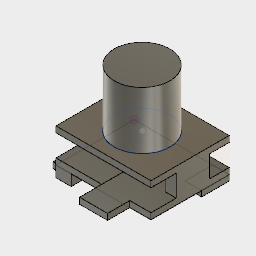
fx805 (Autodesk Fusion 360 design; units mm, degrees)
Autodesk Fusion 360 part; units mm, degrees
sketch "body2" plane through (0, 0, 0) normal (0, 0, 1) x (1, 0, 0)
  line L0 (0, 0) -> (17.1, 0)
  line L1 (17.1, 0) -> (17.1, -14.1)
  line L2 (17.1, -14.1) -> (0, -14.1)
  line L3 (0, -14.1) -> (0, 0)
  line L4 (17.1, 0) -> (14.1, 0)
  line L5 (14.1, 0) -> (14.1, -5)
  line L6 (14.1, -5) -> (17.1, -5)
  line L7 (17.1, -5) -> (17.1, 0)
  dimension "d1" = 17.1
  dimension "d2" = 14.1
  dimension "d19" = 5
  dimension "d20" = 3
  measures "d1" distance of L0.start L0.end
  measures "d2" distance of L0.start L2.end
  measures "d19" distance of L0.end L6.end
  measures "d20" distance of L0.end L4.end
extrude "Extrude1" add sketch "body2" along normal blind 6.1 makes body 1
sketch "body with camera" plane through (0, 0, 6.1) normal (0, 0, 1) x (-1, 0, 0)
  line L0 (0, 14.1) -> (-17.1, 14.1)
  line L1 (-17.1, 14.1) -> (-17.1, 0)
  line L2 (-17.1, 0) -> (0, 0)
  line L3 (0, 0) -> (0, 14.1)
  circle A0 centre (-8.55, 7.1407) radius 5
  dimension "d5" = 10
  measures "d5" diameter of A0
extrude "Extrude2" add sketch "body with camera" along normal blind 10.3 contours A0 bodies 1
sketch "body" plane through (0, 0, 0) normal (0, 0, -1) x (1, 0, 0)
  line L0 (17.1, 14.1) -> (0, 14.1)
  line L1 (0, 14.1) -> (0, 0)
  line L2 (0, 0) -> (17.1, 0)
  line L3 (17.1, 0) -> (17.1, 14.1)
  line L4 (0, 14.1) -> (2.75, 14.1)
  line L5 (2.75, 14.1) -> (2.75, 9.1)
  line L6 (2.75, 9.1) -> (0, 9.1)
  line L7 (0, 9.1) -> (0, 14.1)
  dimension "d8" = 5
  dimension "d9" = 2.75
  measures "d8" distance of L0.end L6.end
  measures "d9" distance of L0.end L4.end
extrude "Extrude3" add sketch "body" along normal blind 2 contours L0 L1 L4 L5 L6 L7 bodies 1
sketch "Sketch6" plane through (0, 0, 0) normal (0, 1, 0) x (-1, 0, 0)
  line L0 (-17.1, 0) -> (0, 0)
  line L1 (0, 0) -> (0, 6.1)
  line L2 (0, 6.1) -> (-17.1, 6.1)
  line L3 (-17.1, 6.1) -> (-17.1, 0)
sketch "Sketch7" plane through (0, 0, 0) normal (-1, 0, 0) x (0, -1, 0)
  line L0 (14.1, -2) -> (14.1, 6.1)
  line L1 (14.1, 6.1) -> (0, 6.1)
  line L2 (0, 6.1) -> (0, 0)
  line L3 (0, 0) -> (9.1, 0)
  line L4 (9.1, 0) -> (9.1, -2)
  line L5 (9.1, -2) -> (14.1, -2)
  line L6 (9.7769, -1.5456) -> (13.3769, -1.5456)
  line L7 (13.3769, -1.5456) -> (13.3769, -0.4527)
  line L8 (13.3769, -0.4527) -> (9.7769, -0.4527)
  line L9 (9.7769, -0.4527) -> (9.7769, -1.5456)
  line L10 (9.7769, -1.5456) -> (13.3769, -0.4527) construction
  line L11 (13.3769, -1.5456) -> (9.7769, -0.4527) construction
  point P0 (11.5769, -0.9991)
extrude "Extrude4" add sketch "Sketch7" along normal blind 1.25 contours L6 L7 L8 L9 bodies 1
sketch "Sketch8" plane through (0, -14.1, 0) normal (0, -1, 0) x (1, 0, 0)
  line L0 (2.75, 0) -> (17.1, 0)
  line L1 (17.1, 0) -> (17.1, 6.1)
  line L2 (17.1, 6.1) -> (0, 6.1)
  line L3 (0, 6.1) -> (0, -2)
  line L4 (0, -2) -> (2.75, -2)
  line L5 (2.75, -2) -> (2.75, 0)
  line L6 (13.3, 0) -> (13.3, 6.1)
  line L7 (13.3, 0) -> (8.25, 0)
  line L8 (8.25, 0) -> (8.25, 1.11)
  line L9 (8.25, 1.11) -> (13.3, 1.11)
  line L10 (13.3, 1.11) -> (13.3, 0)
  dimension "d14" = 3.8
  dimension "d15" = 5.05
  dimension "d16" = 1.11
  measures "d14" distance of L1 L6
  measures "d15" distance of L6.start L7.end
  measures "d16" distance of L6.start L9.end
extrude "Extrude5" add sketch "Sketch8" along normal blind 4 contours L0 L6 L7 L8 L9 L10 bodies 1
extrude "Extrude6" add sketch "body2" against normal blind 1 contours L0 L1 L4 L5 L6 L7 bodies 1
sketch "Sketch9" plane through (0, -14.1, 0) normal (0, -1, 0) x (1, 0, 0)
  line L0 (8.25, 0) -> (8.25, 1.11)
  line L1 (8.25, 1.11) -> (13.3, 1.11)
  line L2 (13.3, 1.11) -> (13.3, 0)
  line L3 (13.3, 0) -> (17.1, 0)
  line L4 (17.1, 0) -> (17.1, 6.1)
  line L5 (17.1, 6.1) -> (0, 6.1)
  line L6 (0, 6.1) -> (0, -2)
  line L7 (0, -2) -> (2.75, -2)
  line L8 (2.75, -2) -> (2.75, 0)
  line L9 (2.75, 0) -> (8.25, 0)
  line L10 (8.25, 1.11) -> (0, 1.1059)
  line L11 (13.3, 1.11) -> (17.642, 1.11)
  line L12 (17.642, 1.11) -> (17.1, 1.11)
  line L13 (0, 5) -> (17.1, 5)
  dimension "d23" = 1.1
  measures "d23" distance of L5 L13
extrude "Extrude7" cut sketch "Sketch9" against normal blind 55 contours L1 L4 L6 L10 L11 L13 bodies 1 makes body 2 at (3.5562, -6.8915, 12.9667)
sketch "Sketch10" plane through (0, 0, 1.11) normal (0, 0, 1) x (-1, 0, 0)
  line L0 (-8.25, 14.1) -> (-8.25, 18.1)
  line L1 (-8.25, 18.1) -> (-13.3, 18.1)
  line L2 (-13.3, 18.1) -> (-13.3, 14.1)
  line L3 (-13.3, 14.1) -> (-17.1, 14.1)
  line L4 (-17.1, 14.1) -> (-17.1, 0)
  line L5 (-17.1, 0) -> (-8.25, 0)
  line L6 (-8.25, 0) -> (-8.25, 14.1)
  line L7 (-17.1, 9.55) -> (-15.1, 9.55)
  line L8 (-15.1, 9.55) -> (-15.1, 3.55)
  line L9 (-15.1, 3.55) -> (-17.1, 3.55)
  line L10 (-17.1, 3.55) -> (-17.1, 9.55)
  line L11 (-17.1, 5) -> (-17.1, 14.1)
  dimension "d26" = 2
  dimension "d27" = 6
  measures "d26" distance of L7.start L7.end
  measures "d27" distance of L7.start L9.end
extrude "Extrude8" add sketch "Sketch10" along normal blind 4 contours L4 L7 L8 L9 L10 L11 bodies 2 1
sketch "Sketch11" plane through (0, 0, 1.11) normal (0, 0, 1) x (-1, 0, 0)
  line L0 (-17.1, 9.55) -> (-15.1, 9.55)
  line L1 (-15.1, 9.55) -> (-15.1, 3.55)
  line L2 (-15.1, 3.55) -> (-17.1, 3.55)
  line L3 (-17.1, 3.55) -> (-17.1, 0)
  line L4 (-17.1, 0) -> (-8.25, 0)
  line L5 (-8.25, 0) -> (-8.25, 14.1) construction
  line L6 (-8.25, 14.1) -> (-8.25, 18.1)
  line L7 (-8.25, 18.1) -> (-13.3, 18.1)
  line L8 (-13.3, 18.1) -> (-13.3, 14.1)
  line L9 (-13.3, 14.1) -> (-17.1, 14.1)
  line L10 (-17.1, 14.1) -> (-17.1, 9.55)
  line L11 (0, 14.1) -> (0, 0)
  line L12 (-15.1, 9.55) -> (0, 9.55) construction
  line L13 (0, 9.1) -> (0, 0)
  line L14 (-15.1, 3.55) -> (0, 3.5539) construction
  line L15 (0, 3.5539) -> (-2.4213, 3.5539)
  line L16 (-2.4213, 3.5539) -> (-2.4213, 9.55)
  line L17 (-2.4213, 9.55) -> (0, 9.55)
  line L18 (0, 9.55) -> (0, 3.5539) construction
extrude "Extrude9" add sketch "Sketch11" along normal blind 4 bodies 2
named bodies: "fx808", "fx808 (1)"
